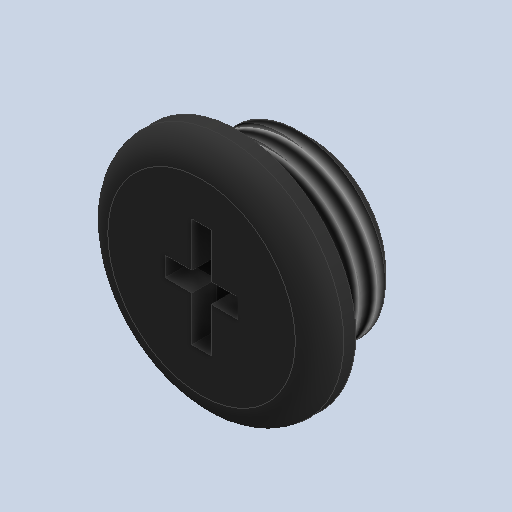
# Autodesk Inventor part: PG9x6mm_Plug
Saved by Autodesk Inventor 2024.2 (Build 282272000, 272)
## iProperties
Created: 2020-07-14
Part Number: PG9x6mm_Plug
Material: Generic
Document SubType Name: Modeling
Designer: CASE-SMALL2
Density: 1 g/cm^3
Appearance: Default
Author: CASE-SMALL2
Autodesk Inventor part; units mm, degrees
ref_plane "YZ Plane" through (0, 0, 0) normal (1, 0, 0) x (0, 1, 0)
ref_plane "XZ Plane" through (0, 0, 0) normal (0, 1, 0) x (-1, 0, 0)
ref_plane "XY Plane" through (0, 0, 0) normal (0, 0, 1) x (1, 0, 0)
sketch "Sketch1" plane through (0, 0, 0) normal (0, 0, 1) x (1, 0, 0)
  circle A0 centre (0, 0) radius 9.75
  dimension "d0" = 19.5
  constraints: 1 centre point, 1 coincident
  measures "d0" diameter of A0
extrude "Extrusion1" add sketch "Sketch1" along normal blind 3
sketch "Sketch2" plane through (0, 0, 0) normal (0, 0, -1) x (-1, 0, 0)
  circle A0 centre (0, 0) radius 7.2
  circle A1 centre (0, 0) radius 4.7
  dimension "d3" = 14.4
  dimension "d4" = 2.5
  constraints: 2 centre point, 2 coincident
  measures "d3" diameter of A0
  measures "d4" radial gap between concentric circles of A0 A1
extrude "Extrusion2" add sketch "Sketch2" along normal blind 6
fillet "Fillet1" radius 2 1 edges at (-9.75, 0, 3)
sketch "Sketch3" plane through (0, 0, 3) normal (0, 0, 1) x (1, 0, 0)
  line L0 (0.8, -4.5) -> (-0.8, -4.5)
  line L1 (-0.8, 4.5) -> (0.8, 4.5)
  line L2 (0.8, -4.5) -> (-0.8, 4.5) construction
  line L3 (-0.8, -4.5) -> (0.8, 4.5) construction
  line L4 (-3, -0.8) -> (-3, 0.8)
  line L5 (3, 0.8) -> (3, -0.8)
  circle A0 centre (0, 0) radius 4.7 projected
  line L6 (3, -0.8) -> (-3, 0.8) construction
  line L7 (-3, -0.8) -> (3, 0.8) construction
  line L8 (3, -0.8) -> (0.8, -0.8)
  line L9 (-0.8, -4.5) -> (-0.8, -0.8)
  line L10 (0.1422, -0.8) -> (-0.1422, -0.8)
  line L11 (-0.8, -0.8) -> (-3, -0.8)
  line L12 (0.8, 0.8) -> (3, 0.8)
  line L13 (-3, 0.8) -> (-0.8, 0.8)
  line L14 (-0.1422, 0.8) -> (0.1422, 0.8)
  line L15 (-0.8, -0.2133) -> (-0.8, 0.2133)
  line L16 (-0.8, 0.8) -> (-0.8, 4.5)
  line L17 (0.8, 4.5) -> (0.8, 0.8)
  line L18 (0.8, 0.2133) -> (0.8, -0.2133)
  line L19 (0.8, -0.8) -> (0.8, -4.5)
  dimension "d8" = 9
  dimension "d9" = 6
  constraints: 40 end point, 20 parallel, 8 point on line, 6 perpendicular, 4 horizontal, 4 midpoint
  measures "d8" distance between parallel lines of L1 L0
  measures "d9" distance between parallel lines of L5 L4
extrude "Extrusion3" cut sketch "Sketch3" against normal blind 2 contours L0 L9 L11 L4 L13 L16 L1 L17 L12 L5 L8 L19
thread "Thread1" size "M15x1.5" class "6g" standard "ANSI Metric M Profile" full length
chamfer "Chamfer1" distance 1 angle 45 1 edges at (7.2, 0, -6)
equation "\"d11\" = d10"
equation "\"d10\" = 1.6"
body "Solid1"
